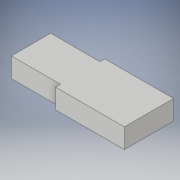
# Autodesk Inventor part: Linear Resistor Post
Saved by Autodesk Inventor 2019 (Build 230136000, 136)
## iProperties
Created: 2019-02-19
Part Number: Linear Resistor Post
Material: Generic
Document SubType Name: Modeling
Designer: Jared
Density: 1 g/cm^3
Appearance: Default
Author: Jared
Autodesk Inventor part; units mm, degrees
ref_plane "YZ Plane" through (0, 0, 0) normal (1, 0, 0) x (0, 1, 0)
ref_plane "XZ Plane" through (0, 0, 0) normal (0, 1, 0) x (-1, 0, 0)
ref_plane "XY Plane" through (0, 0, 0) normal (0, 0, 1) x (1, 0, 0)
sketch "Sketch1" plane through (0, 0, 0) normal (0, 1, 0) x (-1, 0, 0)
  line L0 (0, 0) -> (0, 5)
  line L1 (0, 5) -> (7, 5)
  line L2 (7, 5) -> (7, 4.5)
  line L3 (7, 4.5) -> (12, 4.5)
  line L4 (12, 4.5) -> (12, 0.5)
  line L5 (12, 0.5) -> (7, 0.5)
  line L6 (7, 0.5) -> (7, 0)
  line L7 (7, 0) -> (0, 0)
  dimension "d0" = 5
  dimension "d1" = 7
  dimension "d2" = 0.5
  dimension "d3" = 5
  dimension "d4" = 4
  constraints: 16 end point, 6 perpendicular, 2 point on line, 1 vertical
  measures "d0" distance of L0.start L0.end
  measures "d1" distance of L0.end L1.end
  measures "d2" distance of L1.end L2.end
  measures "d3" distance of L2.end L3.end
  measures "d4" distance of L3.end L4.end
extrude "Extrusion1" add sketch "Sketch1" along normal blind 2
body "Solid1"
